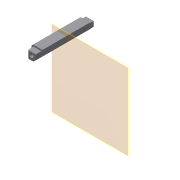
# Autodesk Inventor part: 10_Cube_Side_IM
Saved by Autodesk Inventor 2019 (Build 230136000, 136)
## iProperties
Created: 2021-09-15
Part Number: 10_Cube_Side_IM
Material: Generisch
Document SubType Name: Modeling
Designer: Muriel
Density: 1 g/cm^3
Appearance: Vorgabe
Author: Muriel
Autodesk Inventor part; units mm, degrees
ref_plane "YZ Plane" through (0, 0, 0) normal (1, 0, 0) x (0, 1, 0)
ref_plane "XZ Plane" through (0, 0, 0) normal (0, 1, 0) x (-1, 0, 0)
ref_plane "XY Plane" through (0, 0, 0) normal (0, 0, 1) x (1, 0, 0)
ref_plane "Arbeitsebene1" through (0, 0, 0) normal (0, 0, 1) x (1, 0, 0)
sketch "Skizze1" plane through (0, 0, 0) normal (0, 0, 1) x (1, 0, 0)
  circle A0 centre (-21.2, 21.2) radius 2.75 construction
  arc A1 (-22.85, 24.85) -> (-24.85, 22.85) centre (-22.85, 22.85) ccw projected
  line L0 (-24.85, 22.85) -> (-24.85, 16.97) projected
  line L1 (-24.85, 16.97) -> (-20.75, 16.97) projected
  line L2 (-20.75, 16.97) -> (-19.9236, 17.7964) projected
  arc A2 (-20.2771, 17.65) -> (-19.9236, 17.7964) centre (-20.2771, 18.15) ccw projected
  line L3 (-20.2771, 17.65) -> (-23.25, 17.65) projected
  arc A3 (-23.75, 18.15) -> (-23.25, 17.65) centre (-23.25, 18.15) ccw projected
  line L4 (-23.75, 18.15) -> (-23.75, 23.25) projected
  arc A4 (-23.25, 23.75) -> (-23.75, 23.25) centre (-23.25, 23.25) ccw projected
  line L5 (-23.25, 23.75) -> (-18.15, 23.75) projected
  arc A5 (-17.65, 23.25) -> (-18.15, 23.75) centre (-18.15, 23.25) ccw projected
  line L6 (-17.65, 23.25) -> (-17.65, 20.2771) projected
  arc A6 (-17.7964, 19.9236) -> (-17.65, 20.2771) centre (-18.15, 20.2771) ccw projected
  line L7 (-17.7964, 19.9236) -> (-16.97, 20.75) projected
  line L8 (-16.97, 20.75) -> (-16.97, 24.85) projected
  line L9 (-16.97, 24.85) -> (-22.85, 24.85) projected
  line L10 (-17.7964, 19.9236) -> (-19.9236, 17.7964)
  point P0 (0, 0)
  constraints: 2 end point
extrude "Extrusion1" add sketch "Skizze1" along normal up to surface (17.05 mm away)
sketch "Skizze2" plane through (-22.85, 24.85, 17.05) normal (0, 0, 1) x (1, 0, 0)
  arc A0 (2.5729, -7.2) -> (2.9264, -7.0536) centre (2.5729, -6.7) ccw projected
  line L0 (2.9264, -7.0536) -> (5.0536, -4.9264) projected
  arc A1 (5.0536, -4.9264) -> (5.2, -4.5729) centre (4.7, -4.5729) ccw projected
  line L1 (5.2, -4.5729) -> (5.2, -1.6) projected
  arc A2 (5.2, -1.6) -> (4.7, -1.1) centre (4.7, -1.6) ccw projected
  line L2 (4.7, -1.1) -> (-0.4, -1.1) projected
  arc A3 (-0.4, -1.1) -> (-0.9, -1.6) centre (-0.4, -1.6) ccw projected
  line L3 (-0.9, -1.6) -> (-0.9, -6.7) projected
  arc A4 (-0.9, -6.7) -> (-0.4, -7.2) centre (-0.4, -6.7) ccw projected
  line L4 (-0.4, -7.2) -> (2.5729, -7.2) projected
  circle A5 centre (1.65, -3.65) radius 1.4 projected
  point P0 (22.85, -24.85)
extrude "Extrusion2" add sketch "Skizze2" along normal up to surface (3.7 mm away) draft -2
fillet "Rundung1" radius 0.5 10 edges at (-23.5122, 23.5122, 20.75) (-20.7, 23.6208, 20.75) (-17.8878, 23.5122, 20.75) (-17.7792, 21.7636, 20.75) (-17.8074, 20.1352, 20.75) (-18.9514, 18.9514, 20.75) (-20.1352, 17.8074, 20.75) (-21.7636, 17.7792, 20.75) (-23.5122, 17.8878, 20.75) (-23.6208, 20.7, 20.75)
mirror "Spiegeln1" about plane through (-21.3283, 21.3283, 0) normal (0, 0, -1) of "Extrusion1", "Extrusion2", "Rundung1"
